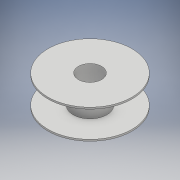
# Autodesk Inventor part: spool
Saved by Autodesk Inventor 2018 (Build 220112000, 112)
## iProperties
Created: 2020-01-12
Part Number: spool
Material: Generic
Document SubType Name: Modeling
Designer: Vinnie Caprarola
Density: 1 g/cm^3
Appearance: Default
Author: Vinnie Caprarola
Autodesk Inventor part; units mm, degrees
ref_plane "YZ Plane" through (0, 0, 0) normal (1, 0, 0) x (0, 1, 0)
ref_plane "XZ Plane" through (0, 0, 0) normal (0, 1, 0) x (-1, 0, 0)
ref_plane "XY Plane" through (0, 0, 0) normal (0, 0, 1) x (1, 0, 0)
sketch "Sketch1" plane through (0, 0, 0) normal (0, 0, 1) x (1, 0, 0)
  circle A0 centre (0, 0) radius 27.5
  circle A1 centre (0, 0) radius 99.5
  circle A2 centre (0, 0) radius 40
  dimension "d0" = 55
  dimension "d1" = 72
  dimension "d2" = 80
  constraints: 3 centre point, 2 coincident
  measures "d0" diameter of A0
  measures "d1" radial gap between concentric circles of A0 A1
  measures "d2" diameter of A2
extrude "Extrusion1" add sketch "Sketch1" along normal blind 66 and the other way blind 4 contours A1 | A2
extrude "Extrusion2" cut sketch "Sketch1" along normal blind 62 contours A1
body "Solid1"
